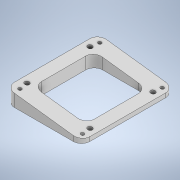
# Autodesk Inventor part: 頸部桌面轉接件
Saved by Autodesk Inventor 2021 (Build 250183000, 183)
## iProperties
Created: 2023-02-10
Part Number: 頸部桌面轉接件
Material: 一般
Document SubType Name: Modeling
Designer: brian
Density: 1 g/cm^3
Appearance: 預設
Author: brian
Autodesk Inventor part; units mm, degrees
ref_plane "YZ Plane" through (0, 0, 0) normal (1, 0, 0) x (0, 1, 0)
ref_plane "XZ Plane" through (0, 0, 0) normal (0, 1, 0) x (-1, 0, 0)
sketch "草圖1" plane through (0, 0, 0) normal (0, 1, 0) x (-1, 0, 0)
  line L0 (90, 110) -> (-90, 110)
  line L1 (-90, 110) -> (-90, -110)
  line L2 (-90, -110) -> (90, -110)
  line L3 (90, -110) -> (90, 110)
  line L4 (90, 110) -> (-90, -110) construction
  line L5 (-90, 110) -> (90, -110) construction
  point P0 (0, 0)
  dimension "d0" = 180
  dimension "d1" = 220
  constraints: 12 end point, 2 midpoint, 2 parallel, 1 horizontal, 1 perpendicular
  measures "d0" distance of L1.end L2.end
  measures "d1" distance of L0.end L1.end
extrude "擠出1" add sketch "草圖1" along normal blind 10
sketch "草圖3" plane through (0, 10, 0) normal (0, 1, 0) x (1, 0, 0)
  line L0 (90, -110) -> (90, 110) projected
  line L1 (90, 110) -> (-90, 110) projected
  line L2 (-90, 110) -> (-90, -110) projected
  line L3 (-90, -110) -> (90, -110) projected
  point P0 (0, 0)
extrude "擠出2" add sketch "草圖3" along normal blind 100
sketch "草圖4" plane through (90, 0, 110) normal (1, 0, 0) x (0, 0, -1)
  line L0 (0, 0) -> (220, 0) projected
  line L1 (220, 0) -> (220, 110) projected
  line L2 (0, 110) -> (220, 110) projected
  line L3 (0, 0) -> (0, 110) projected
  line L4 (0, 0) -> (0, 110) projected
  line L5 (0, 10) -> (220, 10)
  point P0 (110, 0)
  dimension "d7" = 10
  constraints: 2 end point, 2 point on line, 1 perpendicular
  measures "d7" distance between parallel lines of L0 L5
ref_plane "工作平面2" through (90, 10, 110) normal (0.1219, 0.9925, 0) x (0, 0, -1)
split "分割1" plane through (90, 10, 110) removes the side toward (0.1219, 0.9925, 0)
sketch "草圖5" plane through (0, 0, 0) normal (0, -1, 0) x (1, 0, 0)
  line L0 (-75, -75) -> (75, -75) construction
  line L1 (75, -75) -> (75, 75) construction
  line L2 (75, 75) -> (-75, 75) construction
  line L3 (-75, 75) -> (-75, -75) construction
  line L4 (-75, -75) -> (75, 75) construction
  line L5 (75, -75) -> (-75, 75) construction
  point P0 (0, 0)
  dimension "d9" = 150
  dimension "d10" = 150
  constraints: 12 end point, 4 coincident, 2 midpoint, 2 parallel, 1 horizontal, 1 perpendicular
  measures "d9" distance of L2.end L1.end
  measures "d10" distance of L1.end L0.end
hole "孔1" at (-75, 0, -75) at (75, 0, -75) at (75, 0, 75) at (-75, 0, 75) direction (0, 1, 0) diameter 4.2 depth 4
sketch "草圖6" plane through (-75, 4, -75) normal (0, -1, 0) x (1, 0, 0)
  circle A0 centre (0, 150) radius 2.1 projected
  circle A1 centre (150, 150) radius 2.1 projected
  circle A2 centre (150, 0) radius 2.1 projected
  circle A3 centre (0, 0) radius 2.1 projected
  circle A4 centre (0, 0) radius 2.1 projected
  circle A5 centre (150, 0) radius 2.1 projected
  circle A6 centre (0, 150) radius 2.1 projected
  point P0 (75, 75)
  constraints: 4 coincident
hole "孔2" at (-75, 4, -75) at (75, 4, -75) at (75, 4, 75) at (-75, 4, 75) direction (0, 1, 0) diameter 11 end through all
sketch "草圖7" plane through (90, 10, 110) normal (0.1219, 0.9925, 0) x (0.9925, -0.1219, 0)
  line L0 (-163.1105, 15) -> (-13.1105, 15)
  line L1 (-13.1105, 15) -> (-13.1105, 205)
  line L2 (-13.1105, 205) -> (-163.1105, 205)
  line L3 (-163.1105, 205) -> (-163.1105, 15)
  line L4 (-163.1105, 15) -> (-13.1105, 205) construction
  line L5 (-13.1105, 15) -> (-163.1105, 205) construction
  point P0 (-88.1105, 110)
  dimension "d25" = 150
  dimension "d26" = 190
  constraints: 12 end point, 4 coincident, 2 midpoint, 2 parallel, 1 horizontal, 1 perpendicular
  measures "d25" distance of L2.end L1.end
  measures "d26" distance of L1.end L0.end
hole "孔3" at (-71.8947, 29.8782, 95) at (76.9873, 11.5978, 95) at (76.9873, 11.5978, -95) at (-71.8947, 29.8782, -95) direction (-0.1219, -0.9925, 0) diameter 5.5 depth 10 counterbore diameter 8.1 counterbore depth 6
sketch "草圖8" plane through (0, 0, 0) normal (0, -1, 0) x (1, 0, 0)
  line L0 (-62.5, 72.5) -> (62.5, 72.5)
  line L1 (62.5, 72.5) -> (62.5, -72.5)
  line L2 (62.5, -72.5) -> (-62.5, -72.5)
  line L3 (-62.5, -72.5) -> (-62.5, 72.5)
  line L4 (-62.5, 72.5) -> (62.5, -72.5) construction
  line L5 (62.5, 72.5) -> (-62.5, -72.5) construction
  point P0 (0, 0)
  dimension "d34" = 125
  dimension "d35" = 145
  constraints: 12 end point, 2 midpoint, 2 parallel, 1 horizontal, 1 perpendicular
  measures "d34" distance of L1.end L2.end
  measures "d35" distance of L0.end L1.end
extrude "擠出3" cut sketch "草圖8" against normal through all
fillet "圓角2" radius 20 8 edges at (-90, 16.0506, 110) (90, 5, 110) (90, 5, -110) (-90, 16.0506, -110) (-62.5, 14.3623, -72.5) (-62.5, 14.3623, 72.5) (62.5, 6.6883, 72.5) (62.5, 6.6883, -72.5)
equation "\"d9\" = d10"
